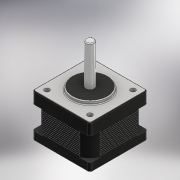
# Autodesk Inventor part: NEMA14
Saved by Autodesk Inventor 2020 (Build 240168000, 168)
## iProperties
Created: 2018-04-20
Part Number: NEMA14
Material: Generic
Document SubType Name: Modeling
Designer: PC  USER
Density: 1 g/cm^3
Appearance: Default
Author: PC  USER
Autodesk Inventor part; units mm, degrees
ref_plane "XY Plane" through (0, 0, 0) normal (0, 0, 1) x (1, 0, 0)
sketch "Sketch1" plane through (0, 0, 0) normal (1, 0, 0) x (0, 1, 0)
  line L0 (17.5, 13) -> (0, 13)
  line L1 (0, -13) -> (17.5, -13)
  line L2 (17.5, -13) -> (17.5, 13)
  line L3 (0, 13) -> (0, -13)
  line L4 (0, 13) -> (11, 13)
  line L5 (11, 13) -> (11, 15)
  line L6 (11, 15) -> (0, 15)
  line L7 (0, 15) -> (0, 13)
  line L8 (0, 15) -> (2.5, 15)
  line L9 (2.5, 15) -> (2.5, 39)
  line L10 (2.5, 39) -> (0, 39)
  line L11 (0, 39) -> (0, 15)
  line L12 (0, 13) -> (-17.5, 13)
  line L13 (-17.5, 13) -> (-17.5, -13)
  line L14 (-17.5, -13) -> (0, -13)
  line L15 (0, -13) -> (0, 13)
  point P0 (0, 0)
  point P1 (17.5, 0)
  dimension "d0" = 26
  dimension "d1" = 2
  dimension "d2" = 24
  dimension "d3" = 17.5
  dimension "d4" = 17.5
  dimension "d5" = 2.5
  dimension "d6" = 11
  constraints: 32 end point, 7 parallel, 4 horizontal, 3 perpendicular, 1 horizontal alignment, 1 midpoint, 1 vertical, 1 vertical alignment
  measures "d0" distance of L1.end L0.start
  measures "d1" distance of L4.end L5.end
  measures "d2" distance of L8.end L9.end
  measures "d3" distance of L1.start L1.end
  measures "d4" distance of L13.end L14.end
  measures "d5" distance of L9.end L10.end
  measures "d6" distance between parallel lines of L7 L5
extrude "Extrusion1" add sketch "Sketch1" along normal mid plane 35 contours L2 L1 L3 L0 | L3 L14 L13 L12
revolve "Revolution1" add sketch "Sketch1" angle 360 about axis through (0, 0, 39) along (0, 0, -1) contours L0 L7 L6 L5 | L11 L10 L9 L6
sketch "Sketch2" plane through (0, 0, 39) normal (0, 0, 1) x (1, 0, 0)
  circle A0 centre (0, 0) radius 2.5 projected
  line L0 (0, 0) -> (0, 2)
  line L1 (0, 2) -> (-2.0798, 2)
  line L2 (0, 2) -> (2.0027, 2)
  arc A1 (2.0027, 2) -> (-2.0798, 2) centre (-0.0386, 0.6448) ccw
  point P0 (0, 0)
  dimension "d10" = 2
  constraints: 6 end point, 2 point on circle, 1 centre point, 1 horizontal, 1 perpendicular, 1 vertical
  measures "d10" distance of L0.start L0.end
extrude "Extrusion2" cut sketch "Sketch2" against normal blind 15 contours L2 L1 A0 | A0 L1 A1 L2 picked at (0.8466, 2.0912)
sketch "Sketch3" plane through (-17.5, -17.5, 13) normal (0, 0, 1) x (1, 0, 0)
  circle A0 centre (17.5, 17.5) radius 11 projected
  line L0 (0, 0) -> (35, 0) projected
  line L1 (35, 35) -> (35, 0) projected
  line L2 (35, 35) -> (0, 35) projected
  line L3 (0, 0) -> (0, 35) projected
  circle A1 centre (30.5, 30.5) radius 1.5
  point P0 (17.5, 17.5)
  dimension "d13" = 3
  dimension "d14" = 13
  dimension "d15" = 13
  constraints: 1 centre point
  measures "d13" diameter of A1
  measures "d14" horizontal distance of A1.centre point (17.5, 17.5)
  measures "d15" horizontal distance of A1.centre point (17.5, 17.5)
extrude "Extrusion3" cut sketch "Sketch3" against normal blind 3.5 contours A1
pattern_circular "Circular Pattern1" count 4 over 360 about axis through (0, 0, -10) along (0, 0, 1) of "Extrusion3"
ref_plane "Work Plane1" through (0, 0, 0) normal (0.7071068, -0.7071068, 0) x (0, 0, -1)
sketch "Sketch4" plane through (0, 0, 0) normal (0.7071068, -0.7071068, 0) x (0, 0, -1)
  line L0 (-13, 24.7487) -> (-13, 0) projected
  line L1 (13, 24.7487) -> (-13, 24.7487) projected
  line L2 (13, 0) -> (13, 24.7487) projected
  line L3 (-13, 0) -> (13, 0) projected
  line L4 (-6, 24.7487) -> (8, 24.7487)
  line L5 (8, 24.7487) -> (8, 20.7487)
  line L6 (8, 20.7487) -> (-6, 20.7487)
  line L7 (-6, 20.7487) -> (-6, 24.7487)
  line L8 (23.4, 0) -> (-49.4, 0) projected
  point P0 (0, 0)
  dimension "d21" = 7
  dimension "d22" = 5
  dimension "d23" = 0
  dimension "d24" = 4
  constraints: 8 end point, 2 parallel, 1 horizontal, 1 perpendicular
  measures "d21" distance between parallel lines of L0 L7
  measures "d22" distance between parallel lines of L2 L5
  measures "d23" distance between parallel lines of L1 L4
  measures "d24" distance between parallel lines of L6 L1
revolve "Revolution2" cut sketch "Sketch4" angle 360 about axis through (0, 0, -10) along (0, 0, 1) contours L1 L5 L6 L7
sketch "Sketch5" plane through (0, 0, 0) normal (1, 0, 0) x (0, 1, 0)
  line L0 (17.5, 6) -> (11.1472, 6) projected
  line L1 (11.1472, 6) -> (11.1472, -8) projected
  line L2 (11.1472, -8) -> (17.5, -8) projected
  line L3 (17.5, -8) -> (17.5, -13) projected
  line L4 (17.5, -13) -> (-17.5, -13) projected
  line L5 (-17.5, -13) -> (-17.5, -8) projected
  line L6 (-17.5, -8) -> (-11.1472, -8) projected
  line L7 (-11.1472, -8) -> (-11.1472, 6) projected
  line L8 (-11.1472, 6) -> (-17.5, 6) projected
  line L9 (-17.5, 6) -> (-17.5, 13) projected
  line L10 (-17.5, 13) -> (17.5, 13) projected
  line L11 (17.5, 13) -> (17.5, 6) projected
  line L12 (-17.5, 6) -> (-17.5, -8) projected
  line L13 (-17.5, 6) -> (-11.1472, 6) projected
  line L14 (-11.1472, -8) -> (-11.1472, 6) projected
  line L15 (-17.5, -8) -> (-11.1472, -8) projected
  line L16 (11.1472, 6) -> (11.1472, -8) projected
  line L17 (11.1472, 6) -> (17.5, 6) projected
  line L18 (17.5, -8) -> (17.5, 6) projected
  line L19 (11.1472, -8) -> (17.5, -8) projected
  line L20 (17.3, 5.1) -> (17.5, 5.1)
  line L21 (17.5, 5.1) -> (17.5, 4.9)
  line L22 (17.5, 4.9) -> (17.3, 4.9)
  line L23 (17.3, 4.9) -> (17.3, 5.1)
  line L24 (17.5, 4.1) -> (17.5, 3.9)
  line L25 (17.3, 4.1) -> (17.5, 4.1)
  line L26 (17.5, 3.9) -> (17.3, 3.9)
  line L27 (17.3, 3.9) -> (17.3, 4.1)
  line L28 (17.5, 3.1) -> (17.5, 2.9)
  line L29 (17.3, 3.1) -> (17.5, 3.1)
  line L30 (17.5, 2.9) -> (17.3, 2.9)
  line L31 (17.3, 2.9) -> (17.3, 3.1)
  line L32 (17.5, 2.1) -> (17.5, 1.9)
  line L33 (17.3, 2.1) -> (17.5, 2.1)
  line L34 (17.5, 1.9) -> (17.3, 1.9)
  line L35 (17.3, 1.9) -> (17.3, 2.1)
  line L36 (17.5, 1.1) -> (17.5, 0.9)
  line L37 (17.3, 1.1) -> (17.5, 1.1)
  line L38 (17.5, 0.9) -> (17.3, 0.9)
  line L39 (17.3, 0.9) -> (17.3, 1.1)
  line L40 (17.5, 0.1) -> (17.5, -0.1)
  line L41 (17.3, 0.1) -> (17.5, 0.1)
  line L42 (17.5, -0.1) -> (17.3, -0.1)
  line L43 (17.3, -0.1) -> (17.3, 0.1)
  line L44 (17.5, -0.9) -> (17.5, -1.1)
  line L45 (17.3, -0.9) -> (17.5, -0.9)
  line L46 (17.5, -1.1) -> (17.3, -1.1)
  line L47 (17.3, -1.1) -> (17.3, -0.9)
  line L48 (17.5, -1.9) -> (17.5, -2.1)
  line L49 (17.3, -1.9) -> (17.5, -1.9)
  line L50 (17.5, -2.1) -> (17.3, -2.1)
  line L51 (17.3, -2.1) -> (17.3, -1.9)
  line L52 (17.5, -2.9) -> (17.5, -3.1)
  line L53 (17.3, -2.9) -> (17.5, -2.9)
  line L54 (17.5, -3.1) -> (17.3, -3.1)
  line L55 (17.3, -3.1) -> (17.3, -2.9)
  line L56 (17.5, -3.9) -> (17.5, -4.1)
  line L57 (17.3, -3.9) -> (17.5, -3.9)
  line L58 (17.5, -4.1) -> (17.3, -4.1)
  line L59 (17.3, -4.1) -> (17.3, -3.9)
  line L60 (17.5, -4.9) -> (17.5, -5.1)
  line L61 (17.3, -4.9) -> (17.5, -4.9)
  line L62 (17.5, -5.1) -> (17.3, -5.1)
  line L63 (17.3, -5.1) -> (17.3, -4.9)
  line L64 (17.5, -5.9) -> (17.5, -6.1)
  line L65 (17.3, -5.9) -> (17.5, -5.9)
  line L66 (17.5, -6.1) -> (17.3, -6.1)
  line L67 (17.3, -6.1) -> (17.3, -5.9)
  line L68 (17.5, -6.9) -> (17.5, -7.1)
  line L69 (17.3, -6.9) -> (17.5, -6.9)
  line L70 (17.5, -7.1) -> (17.3, -7.1)
  line L71 (17.3, -7.1) -> (17.3, -6.9)
  point P0 (0, 0)
  dimension "d26" = 0.2
  dimension "d27" = 0
  dimension "d28" = 0.9
  dimension "d31" = 1
  dimension "d36" = 0.2
  dimension "d37" = 0.9
  constraints: 104 end point, 2 parallel, 1 horizontal, 1 perpendicular, 1 vertical, 96 other
  measures "d26" distance between parallel lines of L18 L23
  measures "d27" distance between parallel lines of L18 L21
  measures "d28" distance between parallel lines of L0 L20
  measures "d31" distance of L20.end L24.start
  measures "d36" distance between parallel lines of L22 L20
  measures "d37" distance between parallel lines of L2 L70
extrude "Extrusion4" cut sketch "Sketch5" along normal mid plane 35 contours L18 L22 L23 L20 | L18 L26 L27 L25 | L70 L71 L69 L18 | L18 L30 L31 L29 | L66 L67 L65 L18 | L18 L34 L35 L33 | L62 L63 L61 L18 | L18 L38 L39 L37 | L58 L59 L57 L18 | L18 L42 L43 L41 | L54 L55 L53 L18 | L18 L46 L47 L45 | L50 L51 L49 L18
pattern_circular "Circular Pattern2" count 4 over 360 about axis through (0, 0, -10) along (0, 0, 1) of "Extrusion4"
fillet "Fillet1" radius 1.5 8 edges at (17.5, 17.5, 9.5) (-17.5, 17.5, 9.5) (-17.5, -17.5, 9.5) (17.5, -17.5, 9.5) (-17.5, 17.5, -10.5) (17.5, 17.5, -10.5) (-17.5, -17.5, -10.5) (17.5, -17.5, -10.5)
fillet "Fillet1" radius 0.5 11 edges at (-17.5, 0, 13) (0, 17.5, 13) (17.5, 0, 13) (0, -17.5, 13) (-17.5, 0, -13) (0, -17.5, -13) (17.5, 0, -13) (0, 17.5, -13) (0, -2.5, 39) (0, -11, 15) (0, -11, 13)
equation "\"d4\" = d3"
body "Solid1"
